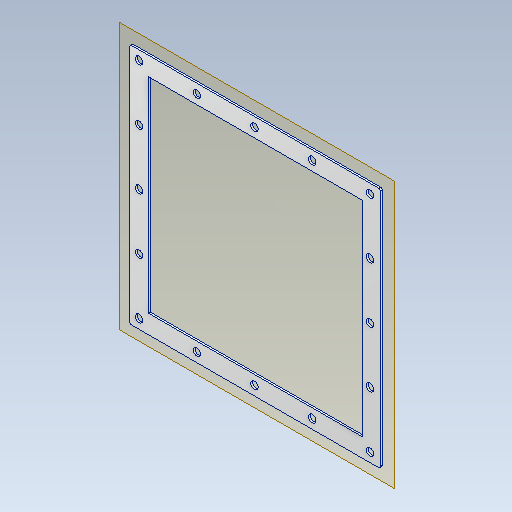
# Autodesk Inventor part: Деталь5_CPY
Saved by Autodesk Inventor 2021 (Build 250183000, 183)
## iProperties
Created: 2020-11-22
Part Number: Деталь5_CPY
Material: Алюминий 6061
Document SubType Name: Modeling
Designer: Тимоха
Mass: 93.8063 g
Surface Area: 404.628 cm^2
Volume: 34.7431 cm^3
Density: 2.7 g/cm^3
Appearance: Алюминий — плоский
Author: Тимоха
Autodesk Inventor part; units mm, degrees
ref_plane "YZ Plane" through (0, 0, 0) normal (1, 0, 0) x (0, 1, 0)
ref_plane "XZ Plane" through (0, 0, 0) normal (0, 1, 0) x (-1, 0, 0)
ref_plane "XY Plane" through (0, 0, 0) normal (0, 0, 1) x (1, 0, 0)
ref_plane "РабПлоскость1" through (0, 0, 0) normal (0, 0, 1) x (1, 0, 0)
sketch "Эскиз1" plane through (0, 0, 0) normal (0, 0, 1) x (1, 0, 0)
  circle A0 centre (123.364, -120) radius 4 projected
  circle A1 centre (61.364, -120) radius 4 projected
  circle A2 centre (-0.636, -120) radius 4 projected
  circle A3 centre (-62.636, -120) radius 4 projected
  circle A4 centre (-124.636, -120) radius 4 projected
  circle A5 centre (123.364, -60) radius 4 projected
  circle A6 centre (-124.636, -60) radius 4 projected
  circle A7 centre (123.364, 0) radius 4 projected
  circle A8 centre (-124.636, 0) radius 4 projected
  circle A9 centre (123.364, 60) radius 4 projected
  circle A10 centre (-124.636, 60) radius 4 projected
  circle A11 centre (123.364, 120) radius 4 projected
  circle A12 centre (61.364, 120) radius 4 projected
  circle A13 centre (-0.636, 120) radius 4 projected
  circle A14 centre (-62.636, 120) radius 4 projected
  circle A15 centre (-124.636, 120) radius 4 projected
  line L0 (115.364, 110) -> (115.364, -110) projected
  line L1 (115.364, -110) -> (-114.636, -110) projected
  line L2 (-114.636, -110) -> (-114.636, 110) projected
  line L3 (-114.636, 110) -> (115.364, 110) projected
  arc A16 (-132.636, 130) -> (-134.636, 128) centre (-132.636, 128) ccw projected
  line L4 (-134.636, 128) -> (-134.636, -128) projected
  arc A17 (-134.636, -128) -> (-132.636, -130) centre (-132.636, -128) ccw projected
  line L5 (-132.636, -130) -> (132.636, -130) projected
  arc A18 (132.636, -130) -> (134.636, -128) centre (132.636, -128) ccw projected
  line L6 (134.636, -128) -> (134.636, 128) projected
  arc A19 (134.636, 128) -> (132.636, 130) centre (132.636, 128) ccw projected
  line L7 (132.636, 130) -> (-132.636, 130) projected
extrude "Выдавливание1" add sketch "Эскиз1" along normal blind 2
